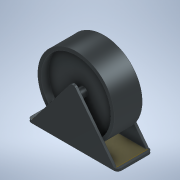
# Autodesk Inventor part: roller_coaster_wheel
Saved by Autodesk Inventor 2020 (Build 240168000, 168)
## iProperties
Created: 2022-09-01
Part Number: roller_coaster_wheel
Material: Iron, Gray
Document SubType Name: Modeling
Designer: Intuito_PC
Density: 7.15 g/cm^3
Appearance: Iron Gray
Author: Intuito_PC
Autodesk Inventor part; units mm, degrees
ref_plane "YZ Plane" through (0, 0, 0) normal (1, 0, 0) x (0, 1, 0)
ref_plane "XY Plane" through (0, 0, 0) normal (0, 0, 1) x (1, 0, 0)
sketch "Sketch1" plane through (0, 0, 0) normal (1, 0, 0) x (0, 1, 0)
  line L0 (-12.5, -12) -> (-9.5, -12)
  line L1 (-9.5, 12) -> (-12.5, 12)
  line L2 (-12.5, 12) -> (-12.5, -12)
  line L3 (-12.5, -12) -> (12.5, 12) construction
  line L4 (12.5, -12) -> (-12.5, 12) construction
  line L5 (20.5, 5.75) -> (-9.5, 5.75)
  line L6 (20.5, -6.75) -> (-9.5, -6.75)
  line L7 (20.5, 5.75) -> (20.5, -6.75)
  line L8 (-9.5, 12) -> (-9.5, 5.75)
  line L9 (-9.5, -6.75) -> (-9.5, -12)
  point P0 (0, 0)
  dimension "d0" = 25
  dimension "d2" = 6.25
  dimension "d3" = 12.5
  dimension "d5" = 24
  dimension "d7" = 3
  dimension "d8" = 3
  dimension "d9" = 30
  constraints: 20 end point, 3 perpendicular, 2 horizontal, 2 midpoint, 1 parallel, 1 vertical
  measures "d0" distance of L1.end L3.end
  measures "d2" distance between parallel lines of L1 L5
  measures "d3" distance between parallel lines of L5 L6
  measures "d5" distance of L1.end L0.start
  measures "d7" distance of L0.start L0.end
  measures "d8" distance of L1.start L1.end
  measures "d9" distance of L5.start L5.end
revolve "Revolution1" add sketch "Sketch1" angle 360 about axis through (0, 20.5, 5.75) along (0, 0, -1)
ref_plane "Work Plane1" through (0, -14.2875, 0) normal (0, 1, 0) x (-1, 0, 0)
sketch "Sketch2" plane through (0, -14.2875, 0) normal (0, 1, 0) x (-1, 0, 0)
  line L0 (38.8032, 14.945) -> (-38.8032, 14.945)
  line L1 (-38.8032, 14.945) -> (-38.8032, -14.945)
  line L2 (-38.8032, -14.945) -> (38.8032, -14.945)
  line L3 (38.8032, -14.945) -> (38.8032, 14.945)
  line L4 (38.8032, 14.945) -> (-38.8032, -14.945) construction
  line L5 (-38.8032, 14.945) -> (38.8032, -14.945) construction
  point P0 (0, 0)
  constraints: 12 end point, 2 midpoint, 2 parallel, 1 horizontal, 1 perpendicular
extrude "Extrusion1" add sketch "Sketch2" against normal blind 2
fillet "Fillet1" radius 3.175 4 edges at (-38.8032, -15.2875, 14.945) (-38.8032, -15.2875, -14.945) (38.8032, -15.2875, 14.945) (38.8032, -15.2875, -14.945)
sketch "Sketch3" plane through (-35.6282, -14.2875, 14.945) normal (0, 0, 1) x (1, 0, 0)
  line L0 (71.2564, 0) -> (74.4314, 0) projected
  line L1 (71.2564, 0) -> (38.1431, 42.9682)
  line L2 (0, -2) -> (0, 0) projected
  line L3 (33.1133, 42.9682) -> (0, 0)
  line L4 (0, 0) -> (71.2564, 0)
  arc A0 (38.1431, 42.9682) -> (33.1133, 42.9682) centre (35.6282, 41.0302) ccw
  point P0 (35.6282, 14.2875)
  dimension "d14" = 3.175
  constraints: 6 end point, 2 point on circle, 2 tangent, 1 centre point, 1 horizontal
  measures "d14" radius of A0
extrude "Extrusion2" add sketch "Sketch3" against normal blind 2
mirror "Mirror1" about plane through (0, 0, 0) normal (0, 0, 1) of "Extrusion2"
sketch "Sketch4" plane through (-35.6282, -16.2875, 14.945) normal (0, 0, 1) x (1, 0, 0)
  circle A0 centre (35.6282, 36.7875) radius 30 projected
  circle A1 centre (35.6282, 36.7875) radius 3.8819
  point P0 (35.6282, 16.2875)
  constraints: 1 centre point, 1 coincident
extrude "Extrusion3" add sketch "Sketch4" against normal blind 28.9875 contours A1
body "Solid1"
